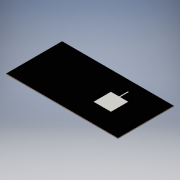
# Autodesk Inventor part: baseField
Saved by Autodesk Inventor 2016 (Build 200138000, 138)
## iProperties
Created: 2016-12-21
Part Number: baseField
Material: Wood (Birch)
Document SubType Name: Modeling
Designer: Naga
Density: 0.55 g/cm^3
Appearance: Birch - Natural Polished
Author: Naga
Autodesk Inventor part; units mm, degrees
ref_plane "YZ Plane" through (0, 0, 0) normal (1, 0, 0) x (0, 1, 0)
ref_plane "XZ Plane" through (0, 0, 0) normal (0, 1, 0) x (-1, 0, 0)
ref_plane "XY Plane" through (0, 0, 0) normal (0, 0, 1) x (1, 0, 0)
sketch "Sketch1" plane through (0, 0, 0) normal (0, 1, 0) x (-1, 0, 0)
  line L0 (0, 0) -> (2438.4, 0)
  line L1 (2438.4, 0) -> (2438.4, -1219.2)
  line L2 (2438.4, -1219.2) -> (0, -1219.2)
  line L3 (0, -1219.2) -> (0, 0)
  dimension "d0" = 2438.4
  dimension "d1" = 1219.2
  constraints: 8 end point, 2 parallel, 1 horizontal, 1 perpendicular
  measures "d0" distance of L1.end L2.end
  measures "d1" distance of L0.end L1.end
extrude "Extrusion1" add sketch "Sketch1" along normal blind 12.7
sketch "Sketch2" plane through (0, 12.7, 0) normal (0, 1, 0) x (1, 0, 0)
  line L0 (0, 0) -> (0, 1219.2) projected
  line L1 (0, 609.6) -> (-38.1, 609.6)
  line L2 (-2438.4, 0) -> (0, 0) projected
  line L3 (-1219.2, 0) -> (-1219.2, 38.1)
  line L4 (-2400.3, 1181.1) -> (-2400.3, 38.1)
  line L5 (-2400.3, 38.1) -> (-38.1, 38.1)
  line L6 (-38.1, 38.1) -> (-38.1, 1181.1)
  line L7 (-38.1, 1181.1) -> (-2400.3, 1181.1)
  line L8 (-2400.3, 1181.1) -> (-38.1, 38.1) construction
  line L9 (-2400.3, 38.1) -> (-38.1, 1181.1) construction
  line L10 (-2438.4, 1219.2) -> (-2438.4, 0) projected
  line L11 (0, 0) -> (-2438.4, 0)
  line L12 (-2438.4, 0) -> (-2438.4, 1219.2)
  line L13 (-2438.4, 1219.2) -> (0, 1219.2)
  line L14 (0, 1219.2) -> (0, 0)
  line L15 (0, 0) -> (-2438.4, 1219.2) construction
  line L16 (-2438.4, 0) -> (0, 1219.2) construction
  line L17 (-38.1, 609.6) -> (-571.5, 609.6)
  line L18 (-571.5, 609.6) -> (-762, 609.6)
  line L19 (-952.5, 419.1) -> (-571.5, 419.1)
  line L20 (-571.5, 419.1) -> (-571.5, 800.1)
  line L21 (-571.5, 800.1) -> (-952.5, 800.1)
  line L22 (-952.5, 800.1) -> (-952.5, 419.1)
  line L23 (-952.5, 419.1) -> (-571.5, 800.1) construction
  line L24 (-571.5, 419.1) -> (-952.5, 800.1) construction
  line L25 (-762, 609.6) -> (-762, 800.1)
  line L26 (-762, 800.1) -> (-762, 990.6)
  line L27 (-762, 800.1) -> (-571.5, 800.1) construction
  line L28 (-762, 895.35) -> (-749.3, 895.35)
  line L29 (-774.7, 800.1) -> (-749.3, 800.1)
  line L30 (-749.3, 800.1) -> (-749.3, 990.6)
  line L31 (-749.3, 990.6) -> (-774.7, 990.6)
  line L32 (-774.7, 990.6) -> (-774.7, 800.1)
  line L33 (-774.7, 800.1) -> (-749.3, 990.6) construction
  line L34 (-749.3, 800.1) -> (-774.7, 990.6) construction
  point P0 (-1219.2, 609.6)
  dimension "d4" = 38.1
  dimension "d5" = 38.1
  dimension "d6" = 533.4
  dimension "d7" = 190.5
  dimension "d8" = 381
  dimension "d9" = 381
  dimension "d10" = 190.5
  dimension "d11" = 90
  dimension "d12" = 12.7
  dimension "d13" = 190.5
  constraints: 64 end point, 12 midpoint, 8 parallel, 7 horizontal, 5 perpendicular, 3 vertical, 1 point on line
  measures "d4" distance of L1.start L1.end
  measures "d5" distance of L3.start L3.end
  measures "d6" distance of L1.end L17.end
  measures "d7" distance of L17.end L18.end
  measures "d8" distance of L21.end L20.end
  measures "d9" distance of L20.end L19.end
  measures "d10" distance of L25.end L26.end
  measures "d11" angle of L27 L26
  measures "d12" distance of L28.start L28.end
  measures "d13" distance of L30.end L29.end
extrude "Extrusion2" add sketch "Sketch2" along normal blind 0.0254 contours L20 L19 L22 L21 L25 L18 | L18 L25 L21 L20 | L26 L28 L30 L21 | L21 L32 L31 L26 | L26 L31 L30 L28
body "Solid1"
